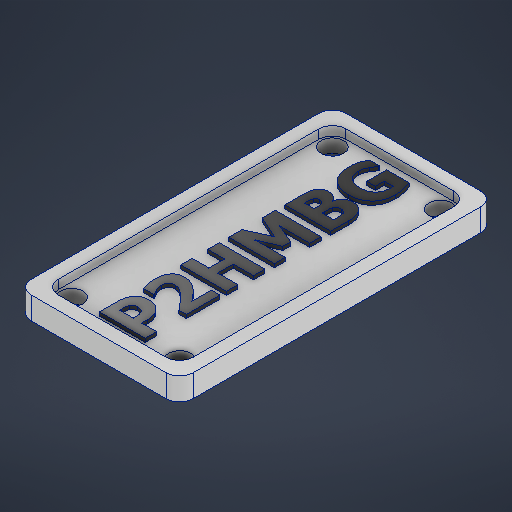
# Autodesk Inventor part: emblem mbg
Saved by Autodesk Inventor 2026.3 (Build 303398000, 398)
## iProperties
Created: 2026-06-09
Part Number: emblem mbg
Material: Aluminum 6061
Document SubType Name: Modeling
Designer: ilyas
Density: 2.7 g/cm^3
Appearance: Aluminum - Flat
Author: ilyas
Autodesk Inventor part; units mm, degrees
ref_plane "YZ Plane" through (0, 0, 0) normal (1, 0, 0) x (0, 1, 0)
ref_plane "XZ Plane" through (0, 0, 0) normal (0, 1, 0) x (-1, 0, 0)
ref_plane "XY Plane" through (0, 0, 0) normal (0, 0, 1) x (1, 0, 0)
sketch "Sketch1" plane through (0, 0, 0) normal (0, 1, 0) x (-1, 0, 0)
  line L0 (-9, 17.5) -> (9, 17.5)
  line L1 (9, 17.5) -> (9, -17.5)
  line L2 (9, -17.5) -> (-9, -17.5)
  line L3 (-9, -17.5) -> (-9, 17.5)
  line L4 (-9, 17.5) -> (9, -17.5) construction
  line L5 (9, 17.5) -> (-9, -17.5) construction
  point P0 (0, 0)
  dimension "d0" = 18
  dimension "d1" = 35
  constraints: 12 end point, 2 midpoint, 2 parallel, 1 horizontal, 1 perpendicular
  measures "d0" distance of L1.end L2.end
  measures "d1" distance of L0.end L1.end
extrude "Extrusion1" add sketch "Sketch1" along normal blind 1.5
sketch "Sketch2" plane through (0, 1.5, 0) normal (0, 1, 0) x (1, 0, 0)
  point P0 (0, 0)
sketch "Sketch3" plane through (0, 1.5, 0) normal (0, 1, 0) x (1, 0, 0)
  line L0 (9, -17.5) -> (-9, -17.5)
  line L1 (-9, -17.5) -> (-9, 17.5)
  line L2 (-9, 17.5) -> (9, 17.5)
  line L3 (9, 17.5) -> (9, -17.5)
  line L4 (9, -17.5) -> (-9, 17.5) construction
  line L5 (-9, -17.5) -> (9, 17.5) construction
  line L6 (-7.5, 16) -> (-7.5, -16)
  line L7 (-7.5, -16) -> (7.5, -16)
  line L8 (7.5, -16) -> (7.5, 16)
  line L9 (7.5, 16) -> (-7.5, 16)
  point P0 (0, 0)
  dimension "d5" = 18
  dimension "d6" = 35
  dimension "d7" = 1.5
  constraints: 20 end point, 4 parallel, 2 midpoint, 2 perpendicular, 1 horizontal, 3 other
  measures "d5" distance of L1.end L2.end
  measures "d6" distance of L0.end L1.end
  measures "d7" distance between parallel lines of L1 L6
emboss "Emboss1" sketch "Sketch3" operation add depth 1 direction (0, -1, 0)
fillet "Fillet2" radius 1.5 4 edges at (9, 1.25, 17.5) (9, 1.25, -17.5) (-9, 1.25, -17.5) (-9, 1.25, 17.5)
fillet "Fillet3" radius 1.5 4 edges at (-7.5, 2, -16) (-7.5, 2, 16) (7.5, 2, 16) (7.5, 2, -16)
sketch "Sketch4" plane through (0, 1.5, 0) normal (0, 1, 0) x (1, 0, 0)
  line L0 (-7.2376, -15.8189) -> (-7.2376, 15.9132) construction
  line L1 (-7.2376, 15.9132) -> (6.9829, 15.9132) construction
  line L2 (6.9829, 15.9132) -> (6.9829, -15.8189) construction
  line L3 (6.9829, -15.8189) -> (-7.2376, -15.8189) construction
  spline S0 degree 2 poles (-1.0701, -10.8271) (-0.716, -10.8271) (-0.0738, -11.0535) (0.1402, -11.2635) knots 0 0 0 1 2 2 2
  spline S1 degree 2 poles (0.1402, -11.2635) (0.2761, -11.3911) (0.4984, -11.704) (0.5766, -11.8892) knots 0 0 0 1 2 2 2
  spline S2 degree 2 poles (0.5766, -11.8892) (0.6548, -12.0786) (0.7454, -12.5191) (0.7454, -12.7908) knots 0 0 0 1 2 2 2
  line L4 (0.7454, -12.7908) -> (0.7454, -13.4577)
  line L5 (0.7454, -13.4577) -> (2.4085, -13.4577)
  line L6 (2.4085, -13.4577) -> (2.4085, -14.7338)
  line L7 (2.4085, -14.7338) -> (-2.6715, -14.7338)
  line L8 (-2.6715, -14.7338) -> (-2.6715, -12.7619)
  spline S3 degree 2 poles (-2.6715, -12.7619) (-2.6715, -12.3256) (-2.5109, -11.6875) (-2.338, -11.4281) knots 0 0 0 1 2 2 2
  spline S4 degree 2 poles (-2.338, -11.4281) (-2.1445, -11.14) (-1.5105, -10.8271) (-1.0701, -10.8271) knots 0 0 0 1 2 2 2
  spline S5 degree 2 poles (-1.0371, -12.1362) (-1.2553, -12.1362) (-1.5641, -12.342) (-1.6217, -12.482) knots 0 0 0 1 2 2 2
  spline S6 degree 2 poles (-1.6217, -12.482) (-1.6999, -12.6631) (-1.7246, -12.9925) (-1.7246, -13.2765) knots 0 0 0 1 2 2 2
  line L9 (-1.7246, -13.2765) -> (-1.7246, -13.4577)
  line L10 (-1.7246, -13.4577) -> (-0.2014, -13.4577)
  line L11 (-0.2014, -13.4577) -> (-0.2014, -13.3671)
  spline S7 degree 2 poles (-0.2014, -13.3671) (-0.2014, -13.1901) (-0.2097, -12.869) (-0.2303, -12.7496) knots 0 0 0 1 2 2 2
  spline S8 degree 2 poles (-0.2303, -12.7496) (-0.2467, -12.6467) (-0.3455, -12.4203) (-0.4073, -12.3585) knots 0 0 0 1 2 2 2
  spline S9 degree 2 poles (-0.4073, -12.3585) (-0.5308, -12.2268) (-0.8066, -12.1362) (-1.0371, -12.1362) knots 0 0 0 1 2 2 2
  line L12 (2.4085, -6.4222) -> (2.4085, -10.1561)
  line L13 (2.4085, -10.1561) -> (1.5811, -10.1561)
  spline S10 degree 2 poles (1.5811, -10.1561) (1.2024, -9.6827) (0.5354, -8.9252) (0.2349, -8.6411) knots 0 0 0 1 2 2 2
  spline S11 degree 2 poles (0.2349, -8.6411) (-0.1562, -8.2665) (-0.7531, -7.9331) (-1.0659, -7.9331) knots 0 0 0 1 2 2 2
  spline S12 degree 2 poles (-1.0659, -7.9331) (-1.42, -7.9331) (-1.7987, -8.3571) (-1.7987, -8.7358) knots 0 0 0 1 2 2 2
  spline S13 degree 2 poles (-1.7987, -8.7358) (-1.7987, -8.9293) (-1.704, -9.2751) (-1.6299, -9.4521) knots 0 0 0 1 2 2 2
  spline S14 degree 2 poles (-1.6299, -9.4521) (-1.5517, -9.625) (-1.387, -9.872) (-1.3459, -9.9338) knots 0 0 0 1 2 2 2
  line L14 (-1.3459, -9.9338) -> (-1.3459, -10.0326)
  line L15 (-1.3459, -10.0326) -> (-2.4533, -10.0326)
  spline S15 degree 2 poles (-2.4533, -10.0326) (-2.5562, -9.8185) (-2.7703, -8.9046) (-2.7703, -8.4806) knots 0 0 0 1 2 2 2
  spline S16 degree 2 poles (-2.7703, -8.4806) (-2.7703, -7.5749) (-1.9634, -6.6445) (-1.2347, -6.6445) knots 0 0 0 1 2 2 2
  spline S17 degree 2 poles (-1.2347, -6.6445) (-0.786, -6.6445) (0.0785, -7.0686) (0.5725, -7.5584) knots 0 0 0 1 2 2 2
  spline S18 degree 2 poles (0.5725, -7.5584) (0.8771, -7.8672) (1.3506, -8.4476) (1.4494, -8.5753) knots 0 0 0 1 2 2 2
  line L16 (1.4494, -8.5753) -> (1.4494, -6.4222)
  line L17 (1.4494, -6.4222) -> (2.4085, -6.4222)
  line L18 (2.4085, -1.4081) -> (2.4085, -2.6843)
  line L19 (2.4085, -2.6843) -> (0.1567, -2.6843)
  line L20 (0.1567, -2.6843) -> (0.1567, -4.4174)
  line L21 (0.1567, -4.4174) -> (2.4085, -4.4174)
  line L22 (2.4085, -4.4174) -> (2.4085, -5.6936)
  line L23 (2.4085, -5.6936) -> (-2.6715, -5.6936)
  line L24 (-2.6715, -5.6936) -> (-2.6715, -4.4174)
  line L25 (-2.6715, -4.4174) -> (-0.8107, -4.4174)
  line L26 (-0.8107, -4.4174) -> (-0.8107, -2.6843)
  line L27 (-0.8107, -2.6843) -> (-2.6715, -2.6843)
  line L28 (-2.6715, -2.6843) -> (-2.6715, -1.4081)
  line L29 (-2.6715, -1.4081) -> (2.4085, -1.4081)
  line L30 (2.4085, 4.8328) -> (2.4085, 3.5649)
  line L31 (2.4085, 3.5649) -> (-0.9589, 3.5649)
  line L32 (-0.9589, 3.5649) -> (1.2147, 2.6427)
  line L33 (1.2147, 2.6427) -> (1.2147, 1.77)
  line L34 (1.2147, 1.77) -> (-0.9589, 0.8478)
  line L35 (-0.9589, 0.8478) -> (2.4085, 0.8478)
  line L36 (2.4085, 0.8478) -> (2.4085, -0.3542)
  line L37 (2.4085, -0.3542) -> (-2.6715, -0.3542)
  line L38 (-2.6715, -0.3542) -> (-2.6715, 1.1154)
  line L39 (-2.6715, 1.1154) -> (-0.1644, 2.2434)
  line L40 (-0.1644, 2.2434) -> (-2.6715, 3.3631)
  line L41 (-2.6715, 3.3631) -> (-2.6715, 4.8328)
  line L42 (-2.6715, 4.8328) -> (2.4085, 4.8328)
  spline S19 degree 2 poles (0.8524, 9.9457) (1.2312, 9.9457) (1.8034, 9.6576) (1.9928, 9.4188) knots 0 0 0 1 2 2 2
  spline S20 degree 2 poles (1.9928, 9.4188) (2.2192, 9.1306) (2.4085, 8.4473) (2.4085, 7.9162) knots 0 0 0 1 2 2 2
  line L43 (2.4085, 7.9162) -> (2.4085, 5.8867)
  line L44 (2.4085, 5.8867) -> (-2.6715, 5.8867)
  line L45 (-2.6715, 5.8867) -> (-2.6715, 7.6774)
  spline S21 degree 2 poles (-2.6715, 7.6774) (-2.6715, 8.2373) (-2.585, 8.8136) (-2.4492, 9.0648) knots 0 0 0 1 2 2 2
  spline S22 degree 2 poles (-2.4492, 9.0648) (-2.3051, 9.3406) (-1.8111, 9.6082) (-1.49, 9.6082) knots 0 0 0 1 2 2 2
  spline S23 degree 2 poles (-1.49, 9.6082) (-1.1195, 9.6082) (-0.539, 9.2377) (-0.4032, 8.9083) knots 0 0 0 1 2 2 2
  line L46 (-0.4032, 8.9083) -> (-0.3785, 8.9083)
  spline S24 degree 2 poles (-0.3785, 8.9083) (-0.2797, 9.3818) (0.3337, 9.9457) (0.8524, 9.9457) knots 0 0 0 1 2 2 2
  spline S25 degree 2 poles (0.8319, 8.6284) (0.5931, 8.6284) (0.3255, 8.439) (0.2555, 8.2497) knots 0 0 0 1 2 2 2
  spline S26 degree 2 poles (0.2555, 8.2497) (0.2102, 8.1344) (0.202, 7.7268) (0.202, 7.3893) knots 0 0 0 1 2 2 2
  line L47 (0.202, 7.3893) -> (0.202, 7.1546)
  line L48 (0.202, 7.1546) -> (1.4823, 7.1546)
  line L49 (1.4823, 7.1546) -> (1.4823, 7.2246)
  spline S27 degree 2 poles (1.4823, 7.2246) (1.4823, 7.7186) (1.4699, 8.0973) (1.3835, 8.2949) knots 0 0 0 1 2 2 2
  spline S28 degree 2 poles (1.3835, 8.2949) (1.3053, 8.4678) (1.0171, 8.6284) (0.8319, 8.6284) knots 0 0 0 1 2 2 2
  spline S29 degree 2 poles (-1.2388, 8.3114) (-1.3623, 8.3114) (-1.6217, 8.1838) (-1.6793, 8.0521) knots 0 0 0 1 2 2 2
  spline S30 degree 2 poles (-1.6793, 8.0521) (-1.737, 7.9286) (-1.7452, 7.5828) (-1.7452, 7.2411) knots 0 0 0 1 2 2 2
  line L50 (-1.7452, 7.2411) -> (-1.7452, 7.1546)
  line L51 (-1.7452, 7.1546) -> (-0.6666, 7.1546)
  line L52 (-0.6666, 7.1546) -> (-0.6666, 7.3152)
  spline S31 degree 2 poles (-0.6666, 7.3152) (-0.6666, 7.6404) (-0.679, 7.9039) (-0.7448, 8.0438) knots 0 0 0 1 2 2 2
  spline S32 degree 2 poles (-0.7448, 8.0438) (-0.8189, 8.1961) (-1.0701, 8.3114) (-1.2388, 8.3114) knots 0 0 0 1 2 2 2
  spline S33 degree 2 poles (2.1204, 14.9187) (2.2562, 14.5853) (2.5156, 13.519) (2.5156, 13.0003) knots 0 0 0 1 2 2 2
  spline S34 degree 2 poles (2.5156, 13.0003) (2.5156, 11.8024) (1.1324, 10.3821) (-0.1356, 10.3821) knots 0 0 0 1 2 2 2
  spline S35 degree 2 poles (-0.1356, 10.3821) (-1.3294, 10.3821) (-2.7703, 11.8024) (-2.7703, 13.0374) knots 0 0 0 1 2 2 2
  spline S36 degree 2 poles (-2.7703, 13.0374) (-2.7703, 13.6755) (-2.5274, 14.4741) (-2.3215, 14.8981) knots 0 0 0 1 2 2 2
  line L53 (-2.3215, 14.8981) -> (-1.1277, 14.8981)
  line L54 (-1.1277, 14.8981) -> (-1.1277, 14.7829)
  spline S37 degree 2 poles (-1.1277, 14.7829) (-1.1977, 14.6923) (-1.4653, 14.3465) (-1.5558, 14.1818) knots 0 0 0 1 2 2 2
  spline S38 degree 2 poles (-1.5558, 14.1818) (-1.667, 13.9925) (-1.8234, 13.4902) (-1.8234, 13.2103) knots 0 0 0 1 2 2 2
  spline S39 degree 2 poles (-1.8234, 13.2103) (-1.8234, 12.8851) (-1.6176, 12.3458) (-1.4076, 12.1358) knots 0 0 0 1 2 2 2
  spline S40 degree 2 poles (-1.4076, 12.1358) (-1.2018, 11.9341) (-0.5719, 11.6995) (-0.1562, 11.6995) knots 0 0 0 1 2 2 2
  spline S41 degree 2 poles (-0.1562, 11.6995) (0.7331, 11.6995) (1.5811, 12.5928) (1.5811, 13.3626) knots 0 0 0 1 2 2 2
  spline S42 degree 2 poles (1.5811, 13.3626) (1.5811, 13.4326) (1.5729, 13.6137) (1.5687, 13.6837) knots 0 0 0 1 2 2 2
  line L55 (1.5687, 13.6837) -> (0.5684, 13.6837)
  line L56 (0.5684, 13.6837) -> (0.5684, 12.6998)
  line L57 (0.5684, 12.6998) -> (-0.3826, 12.6998)
  line L58 (-0.3826, 12.6998) -> (-0.3826, 14.9187)
  line L59 (-0.3826, 14.9187) -> (2.1204, 14.9187)
  point P0 (0, 0)
  constraints: 2 other
emboss "Emboss2" sketch "Sketch4" operation add depth 0.4 direction (0, -1, 0)
sketch "Sketch5" plane through (0, 1.5, 0) normal (0, 1, 0) x (1, 0, 0)
  arc A0 (-7.5, -14.5) -> (-6, -16) centre (-6, -14.5) ccw projected
  arc A1 (-6, 16) -> (-7.5, 14.5) centre (-6, 14.5) ccw projected
  arc A2 (7.5, 14.5) -> (6, 16) centre (6, 14.5) ccw projected
  arc A3 (6, -16) -> (7.5, -14.5) centre (6, -14.5) ccw projected
  point P0 (0, 0)
  constraints: 4 coincident
hole "Hole1" at (-6, 1.5, 14.5) at (6, 1.5, 14.5) at (6, 1.5, -14.5) at (-6, 1.5, -14.5) direction (0, -1, 0) diameter 2.5 end through all
body "Solid1"
